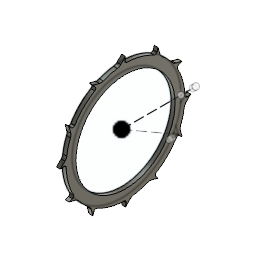
Bidirectional Cleat with Parameters (Autodesk Fusion 360 design; units mm, degrees)
Autodesk Fusion 360 part; units mm, degrees
sketch "Sketch1" plane through (0, 0, 0) normal (1, 0, 0) x (0, 1, 0)
  circle A0 centre (0, 0) radius 25
  circle A1 centre (0, 0) radius 30
  line L0 (0, 0) -> (30, 0) construction
  line L1 (30, 0) -> (33, 0) construction
  line L2 (33, 0) -> (29.9953, -0.5298)
  line L3 (33, 0) -> (36.051, 0) construction
  line L4 (0, 0) -> (30, 0) construction
  line L5 (0, 0) -> (25.9808, -15) construction
  line L6 (0, 0) -> (30, 0) construction
  line L7 (25.9808, -15) -> (28.5788, -16.5) construction
  line L8 (28.5788, -16.5) -> (26.2416, -14.5388)
  line L9 (28.5788, -16.5) -> (25.5278, -16.5) construction
  line L10 (28.5788, -16.5) -> (27.4194, -12.1728)
  line L11 (28.5788, -16.5) -> (24.099, -16.5) construction
  line L12 (33, 0) -> (29.8323, -3.1677)
  line L13 (33, 0) -> (37.4798, 0) construction
  dimension "d7" = 50
  dimension "d8" = 60
  dimension "d10" = 3
  dimension "d11" = 170
  dimension "d27" = 30
  dimension "d28" = 3
  dimension "d29" = 40
  dimension "d30" = 75
  dimension "d31" = 135
  constraint coincident A0.centre A1.centre
  constraint concentric A0 A1
  constraint coincident A1 L0.end
  constraint horizontal L0
  constraint parallel L0 L1
  constraint horizontal L3
  constraint coincident A1 L2.end
  constraint horizontal L4
  constraint horizontal L6
  constraint coincident A1 L5.end
  constraint parallel L5 L7
  constraint horizontal L9
  constraint coincident A1 L8.end
  constraint horizontal L11
  constraint coincident A1 L10.end
  constraint horizontal L13
  constraint coincident A1 L12.end
  measures "d7" diameter of A0
  measures "d8" diameter of A1
  measures "d10" distance of L0.end L1.end
  measures "d11" angle of L2 L3
  measures "d27" angle of L5 L6
  measures "d28" distance of L5.end L7.end
  measures "d29" angle of L8 L9
  measures "d30" angle of L10 L11
  measures "d31" angle of L12 L13
extrude "Extrude1" add sketch "Sketch1" along normal blind 2 contours A1
extrude "Extrude2" add sketch "Sketch1" along normal blind 2 contours A1 L8 L10 | A1 L2 L12
fillet "Fillet1" radius 1 2 edges at (1, 29.9953, -0.5298) (1, 26.2416, -14.5388)
fillet "Fillet1" radius 3 2 edges at (1, 29.8323, -3.1677) (1, 27.4194, -12.1728)
pattern_circular "C-Pattern1" count 6 over 360 about axis through (1.75, 0, 0) along (1, 0, 0) of "Extrude2", "Fillet1"
equation "inner_diameter = 50 mm"
equation "outer_diameter = 60 mm"
equation "spike_length = 3 mm"
equation "spike_pairs = 6"
equation "rake = 10 deg"
equation "relief = 45 deg"
equation "d7 = inner_diameter"
equation "d8 = outer_diameter"
equation "d10 = spike_length"
equation "d11 = 180 deg - rake"
equation "thickness = 2 mm"
equation "d14 = thickness"
equation "rake_fillet = 1 mm"
equation "relief_fillet = 3 mm"
equation "d21 = rake_fillet"
equation "d24 = spike_pairs"
equation "d27 = ( 180 / spike_pairs ) * 1 deg"
equation "d28 = spike_length"
equation "d29 = ( 180 / spike_pairs ) * 1 deg + rake"
equation "d30 = ( 180 / spike_pairs ) * 1 deg + relief"
equation "d31 = 180 deg - relief"
equation "d33 = relief_fillet"
